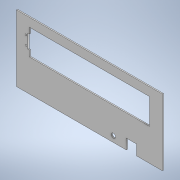
# Autodesk Inventor part: 220228 Back Piece
Saved by Autodesk Inventor 2022 (Build 260153000, 153)
## iProperties
Created: 2022-02-28
Part Number: 220228 Back Piece
Material: Generic
Document SubType Name: Modeling
Designer: josephinew
Density: 1 g/cm^3
Appearance: Default
Author: josephinew
Autodesk Inventor part; units mm, degrees
ref_plane "YZ Plane" through (0, 0, 0) normal (1, 0, 0) x (0, 1, 0)
ref_plane "XZ Plane" through (0, 0, 0) normal (0, 1, 0) x (-1, 0, 0)
ref_plane "XY Plane" through (0, 0, 0) normal (0, 0, 1) x (1, 0, 0)
sketch "Sketch1" plane through (0, 0, 0) normal (0, 0, 1) x (1, 0, 0)
  line L0 (0, 0) -> (431.8, 0)
  line L1 (431.8, 0) -> (431.8, 196.85)
  line L2 (431.8, 196.85) -> (0, 196.85)
  line L3 (0, 196.85) -> (0, 0)
  line L4 (431.8, 0) -> (330.2, 0)
  line L5 (330.2, 0) -> (287.02, 0)
  line L6 (325.12, 0) -> (325.12, 30.48)
  line L7 (325.12, 30.48) -> (355.6, 30.48)
  line L8 (355.6, 30.48) -> (355.6, 0)
  line L9 (38.1, 171.45) -> (393.7, 171.45)
  line L10 (393.7, 171.45) -> (393.7, 95.25)
  line L11 (393.7, 95.25) -> (38.1, 95.25)
  line L12 (38.1, 95.25) -> (38.1, 171.45)
  line L13 (0, 196.85) -> (25.4, 196.85)
  line L14 (431.8, 196.85) -> (406.4, 196.85)
  line L15 (0, 196.85) -> (38.1, 196.85)
  line L16 (38.1, 196.85) -> (38.1, 171.45)
  line L17 (431.8, 0) -> (355.6, 0)
  line L18 (355.6, 0) -> (330.2, 0)
  line L19 (325.12, 0) -> (287.02, 0)
  point P0 (325.12, 0)
  dimension "d0" = 431.8
  dimension "d5" = 30.48
  dimension "d6" = 30.48
  dimension "d7" = 355.6
  dimension "d8" = 76.2
  dimension "d9" = 25.4
  dimension "d15" = 38.1
  dimension "d16" = 76.2
  dimension "d18" = 38.1
  constraints: 40 end point, 6 parallel, 4 perpendicular, 4 point on line, 3 horizontal, 2 collinear
  measures "d0" distance of L2.end L1.end
  measures "d5" distance of L6.end L7.end
  measures "d6" distance of L6.start L6.end
  measures "d7" distance of L10.end L11.end
  measures "d8" distance of L9.end L10.end
  measures "d9" distance of L2.end L13.end
  measures "d15" distance of L2.end L15.end
  measures "d16" distance of L0.end L17.end
  measures "d18" distance of L6.start L5.end
extrude "Extrusion1" add sketch "Sketch1" along normal blind 3.175 contours L3 L2 L1 L0 L8 L7 L6
sketch "Sketch2" plane through (0, 0, 3.175) normal (0, 0, 1) x (1, 0, 0)
  line L0 (0, 0) -> (325.12, 0) projected
  circle A0 centre (27.94, 120.142) radius 2.54
  circle A1 centre (27.94, 146.558) radius 2.54
  line L1 (38.1, 171.45) -> (393.7, 171.45) projected
  line L2 (38.1, 171.45) -> (38.1, 152.4)
  line L3 (38.1, 95.25) -> (38.1, 171.45) projected
  line L4 (38.1, 95.25) -> (38.1, 171.45) projected
  line L5 (38.1, 171.45) -> (38.1, 133.35)
  line L6 (287.02, 0) -> (287.02, 17.78)
  circle A2 centre (287.02, 17.78) radius 6.35
  dimension "d44" = 17.78
  dimension "d45" = 12.7
  constraints: 6 end point, 3 centre point, 2 point on line, 1 coincident, 1 midpoint, 1 vertical
  measures "d44" distance of L6.start L6.end
  measures "d45" diameter of A2
extrude "Extrusion2" cut sketch "Sketch2" against normal blind 25.4
sketch "Sketch4" plane through (0, 0, 3.175) normal (0, 0, 1) x (1, 0, 0)
  circle A0 centre (27.94, 146.558) radius 2.54 projected
  line L0 (27.94, 146.558) -> (27.94, 152.4)
  line L1 (27.94, 152.4) -> (38.1, 152.4)
  line L2 (38.1, 95.25) -> (38.1, 171.45) projected
  line L3 (38.1, 152.4) -> (38.1, 114.3)
  line L4 (38.1, 114.3) -> (27.94, 114.3)
  circle A1 centre (27.94, 120.142) radius 2.54 projected
  line L5 (27.94, 114.3) -> (27.94, 120.142)
  line L6 (38.1, 152.4) -> (35.56, 152.4)
  line L7 (35.56, 152.4) -> (35.56, 114.3)
  point P0 (0, 0)
  dimension "d30" = 5.842
  dimension "d31" = 38.1
  dimension "d32" = 2.54
  constraints: 14 end point, 5 perpendicular, 4 point on line, 1 vertical
  measures "d30" distance of L0.start L0.end
  measures "d31" distance of L1.end L3.end
  measures "d32" distance of L1.end L6.end
extrude "Extrusion3" cut sketch "Sketch4" against normal blind 25.4 contours L1 L2 L4 L7
sketch "Sketch6" plane through (0, 0, 3.175) normal (0, 0, 1) x (1, 0, 0)
  line L0 (38.1, 152.4) -> (38.1, 171.45) projected
  line L1 (35.56, 153.9875) -> (38.1, 153.9875)
  line L2 (38.1, 153.9875) -> (38.1, 112.7125)
  line L3 (38.1, 112.7125) -> (33.7312, 112.7125)
  line L4 (33.7312, 112.7125) -> (33.7312, 153.9875)
  line L5 (33.7312, 153.9875) -> (35.56, 153.9875)
  point P0 (0, 0)
  dimension "d40" = 41.275
  dimension "d41" = 4.3688
  constraints: 10 end point, 3 perpendicular, 1 point on line, 1 vertical
  measures "d40" distance of L1.end L2.end
  measures "d41" distance of L2.end L3.end
extrude "Extrusion4" cut sketch "Sketch6" against normal blind 25.4
body "Solid1"
